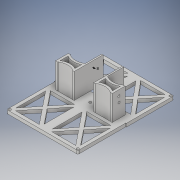
# Autodesk Inventor part: 4 Tape Measure Holder 2 Lid
Saved by Autodesk Inventor 2019 (Build 230136000, 136)
## iProperties
Created: 2019-01-05
Part Number: 4 Tape Measure Holder 2 Lid
Material: Generic
Document SubType Name: Modeling
Designer: ashle
Density: 1 g/cm^3
Appearance: Default
sut: 4.300 mm
TMROL: 45.000 mm
AW: 4.000 mm
WD: 50.000 mm
WW: 20.000 mm
sh: 4.000 mm
BSHH: 10.000 mm
Author: ashle
Autodesk Inventor part; units mm, degrees
ref_plane "YZ Plane" through (0, 0, 0) normal (1, 0, 0) x (0, 1, 0)
ref_plane "XZ Plane" through (0, 0, 0) normal (0, 1, 0) x (-1, 0, 0)
ref_plane "XY Plane" through (0, 0, 0) normal (0, 0, 1) x (1, 0, 0)
sketch "Main Body Sketch" plane through (0, 0, 0) normal (0, 1, 0) x (-1, 0, 0)
  line L0 (162.9728, 0) -> (-170.7717, 0) construction
  line L1 (0, -112.4599) -> (0, 110.3364) construction
  line L2 (65, -85.25) -> (-65, -85.25)
  line L3 (-65, -85.25) -> (-65, 0)
  line L4 (-65, 0) -> (65, 0)
  line L5 (65, 0) -> (65, -85.25)
  line L6 (64, 0) -> (-64, 0)
  line L7 (-64, 0) -> (-64, 86.25)
  line L8 (-64, 86.25) -> (64, 86.25)
  line L9 (64, 86.25) -> (64, 0)
  line L10 (7.5, -85.25) -> (-7.5, -85.25)
  line L11 (-7.5, -85.25) -> (-7.5, 86.25) construction
  line L12 (-7.5, 86.25) -> (7.5, 86.25)
  line L13 (7.5, 86.25) -> (7.5, -85.25) construction
  line L14 (65, -11.5) -> (-65, -11.5) construction
  line L15 (-65, -11.5) -> (-65, 0) construction
  line L16 (-65, 0) -> (65, 0) construction
  line L17 (65, 0) -> (65, -11.5) construction
  line L18 (64, 0) -> (-64, 0)
  line L19 (-64, 0) -> (-64, 11.5) construction
  line L20 (-64, 11.5) -> (64, 11.5) construction
  line L21 (64, 11.5) -> (64, 0) construction
  line L22 (59, -79.25) -> (7.5, -79.25) construction
  line L23 (7.5, -79.25) -> (7.5, -17.5) construction
  line L24 (7.5, -17.5) -> (59, -17.5) construction
  line L25 (59, -17.5) -> (59, -79.25) construction
  line L26 (-7.5, -79.25) -> (-59, -79.25) construction
  line L27 (-59, -79.25) -> (-59, -17.5) construction
  line L28 (-59, -17.5) -> (-7.5, -17.5) construction
  line L29 (-7.5, -17.5) -> (-7.5, -79.25) construction
  line L30 (58, 17.5) -> (7.5, 17.5) construction
  line L31 (7.5, 17.5) -> (7.5, 80.25) construction
  line L32 (7.5, 80.25) -> (58, 80.25) construction
  line L33 (58, 80.25) -> (58, 17.5) construction
  line L34 (-7.5, 17.5) -> (-58, 17.5) construction
  line L35 (-58, 17.5) -> (-58, 80.25) construction
  line L36 (-58, 80.25) -> (-7.5, 80.25) construction
  line L37 (-7.5, 80.25) -> (-7.5, 17.5) construction
  line L38 (59, -79.25) -> (7.5, -17.5) construction
  line L39 (7.5, -79.25) -> (59, -17.5) construction
  line L40 (58, 17.5) -> (7.5, 80.25) construction
  line L41 (7.5, 17.5) -> (58, 80.25) construction
  line L42 (55.6629, 15.6191) -> (60.3371, 19.3809) construction
  line L43 (60.3371, 19.3809) -> (9.8371, 82.1309) construction
  line L44 (9.8371, 82.1309) -> (5.1629, 78.3691) construction
  line L45 (5.1629, 78.3691) -> (55.6629, 15.6191) construction
  line L46 (61.3039, -77.3285) -> (56.6961, -81.1715) construction
  line L47 (56.6961, -81.1715) -> (5.1961, -19.4215) construction
  line L48 (5.1961, -19.4215) -> (9.8039, -15.5785) construction
  line L49 (9.8039, -15.5785) -> (61.3039, -77.3285) construction
  line L50 (9.8039, -81.1715) -> (5.1961, -77.3285) construction
  line L51 (5.1961, -77.3285) -> (56.6961, -15.5785) construction
  line L52 (56.6961, -15.5785) -> (61.3039, -19.4215) construction
  line L53 (61.3039, -19.4215) -> (9.8039, -81.1715) construction
  line L54 (9.8371, 15.6191) -> (5.1629, 19.3809) construction
  line L55 (5.1629, 19.3809) -> (55.6629, 82.1309) construction
  line L56 (55.6629, 82.1309) -> (60.3371, 78.3691) construction
  line L57 (60.3371, 78.3691) -> (9.8371, 15.6191) construction
  line L58 (33.25, -43.6911) -> (55.0936, -17.5)
  line L59 (55.0936, -17.5) -> (11.4064, -17.5)
  line L60 (11.4064, -17.5) -> (33.25, -43.6911)
  line L61 (54.1491, 17.5) -> (32.75, 44.09)
  line L62 (32.75, 44.09) -> (11.3509, 17.5)
  line L63 (11.3509, 17.5) -> (54.1491, 17.5)
  line L64 (58, 22.285) -> (58, 75.465)
  line L65 (58, 75.465) -> (36.6009, 48.875)
  line L66 (36.6009, 48.875) -> (58, 22.285)
  line L67 (32.75, 53.66) -> (54.1491, 80.25)
  line L68 (54.1491, 80.25) -> (11.3509, 80.25)
  line L69 (11.3509, 80.25) -> (32.75, 53.66)
  line L70 (7.5, 22.285) -> (28.8991, 48.875)
  line L71 (28.8991, 48.875) -> (7.5, 75.465)
  line L72 (7.5, 75.465) -> (7.5, 22.285)
  line L73 (59, -74.5661) -> (59, -22.1839)
  line L74 (59, -22.1839) -> (37.1564, -48.375)
  line L75 (37.1564, -48.375) -> (59, -74.5661)
  line L76 (55.0936, -79.25) -> (33.25, -53.0589)
  line L77 (33.25, -53.0589) -> (11.4064, -79.25)
  line L78 (11.4064, -79.25) -> (55.0936, -79.25)
  line L79 (7.5, -74.5661) -> (29.3436, -48.375)
  line L80 (29.3436, -48.375) -> (7.5, -22.1839)
  line L81 (7.5, -22.1839) -> (7.5, -74.5661)
  line L82 (-59, -79.25) -> (-7.5, -79.25) construction
  line L83 (-7.5, -79.25) -> (-7.5, -17.5) construction
  line L84 (-7.5, -17.5) -> (-59, -17.5) construction
  line L85 (-59, -17.5) -> (-59, -79.25) construction
  line L86 (-59, -79.25) -> (-7.5, -17.5) construction
  line L87 (-7.5, -79.25) -> (-59, -17.5) construction
  line L88 (-61.3039, -77.3285) -> (-56.6961, -81.1715) construction
  line L89 (-56.6961, -81.1715) -> (-5.1961, -19.4215) construction
  line L90 (-5.1961, -19.4215) -> (-9.8039, -15.5785) construction
  line L91 (-9.8039, -15.5785) -> (-61.3039, -77.3285) construction
  line L92 (-9.8039, -81.1715) -> (-5.1961, -77.3285) construction
  line L93 (-5.1961, -77.3285) -> (-56.6961, -15.5785) construction
  line L94 (-56.6961, -15.5785) -> (-61.3039, -19.4215) construction
  line L95 (-61.3039, -19.4215) -> (-9.8039, -81.1715) construction
  line L96 (-33.25, -43.6911) -> (-55.0936, -17.5)
  line L97 (-55.0936, -17.5) -> (-11.4064, -17.5)
  line L98 (-11.4064, -17.5) -> (-33.25, -43.6911)
  line L99 (-59, -74.5661) -> (-59, -22.1839)
  line L100 (-59, -22.1839) -> (-37.1564, -48.375)
  line L101 (-37.1564, -48.375) -> (-59, -74.5661)
  line L102 (-55.0936, -79.25) -> (-33.25, -53.0589)
  line L103 (-33.25, -53.0589) -> (-11.4064, -79.25)
  line L104 (-11.4064, -79.25) -> (-55.0936, -79.25)
  line L105 (-7.5, -74.5661) -> (-29.3436, -48.375)
  line L106 (-29.3436, -48.375) -> (-7.5, -22.1839)
  line L107 (-7.5, -22.1839) -> (-7.5, -74.5661)
  line L108 (-58, 17.5) -> (-7.5, 17.5) construction
  line L109 (-7.5, 17.5) -> (-7.5, 80.25) construction
  line L110 (-7.5, 80.25) -> (-58, 80.25) construction
  line L111 (-58, 80.25) -> (-58, 17.5) construction
  line L112 (-58, 17.5) -> (-7.5, 80.25) construction
  line L113 (-7.5, 17.5) -> (-58, 80.25) construction
  line L114 (-55.6629, 15.6191) -> (-60.3371, 19.3809) construction
  line L115 (-60.3371, 19.3809) -> (-9.8371, 82.1309) construction
  line L116 (-9.8371, 82.1309) -> (-5.1629, 78.3691) construction
  line L117 (-5.1629, 78.3691) -> (-55.6629, 15.6191) construction
  line L118 (-9.8371, 15.6191) -> (-5.1629, 19.3809) construction
  line L119 (-5.1629, 19.3809) -> (-55.6629, 82.1309) construction
  line L120 (-55.6629, 82.1309) -> (-60.3371, 78.3691) construction
  line L121 (-60.3371, 78.3691) -> (-9.8371, 15.6191) construction
  line L122 (-54.1491, 17.5) -> (-32.75, 44.09)
  line L123 (-32.75, 44.09) -> (-11.3509, 17.5)
  line L124 (-11.3509, 17.5) -> (-54.1491, 17.5)
  line L125 (-58, 22.285) -> (-58, 75.465)
  line L126 (-58, 75.465) -> (-36.6009, 48.875)
  line L127 (-36.6009, 48.875) -> (-58, 22.285)
  line L128 (-32.75, 53.66) -> (-54.1491, 80.25)
  line L129 (-54.1491, 80.25) -> (-11.3509, 80.25)
  line L130 (-11.3509, 80.25) -> (-32.75, 53.66)
  line L131 (-7.5, 22.285) -> (-28.8991, 48.875)
  line L132 (-28.8991, 48.875) -> (-7.5, 75.465)
  line L133 (-7.5, 75.465) -> (-7.5, 22.285)
  line L134 (71.3038, -11) -> (3.6263, -11) construction
  line L135 (71.3038, -7) -> (3.6263, -7) construction
  line L136 (47, -13.6904) -> (47, -1.8887) construction
  line L137 (20, -13.6904) -> (20, -1.8887) construction
  line L138 (47, -11.5) -> (20, -11.5)
  line L139 (20, -11.5) -> (20, -11)
  line L140 (47, -11.5) -> (47, -11)
  line L141 (33.5, -14.616) -> (33.5, -1.8887) construction
  arc A0 (47, -11) -> (20, -11) centre (33.5, -31.7812) ccw
  line L142 (-47, -13.6904) -> (-47, -1.8887) construction
  line L143 (-20, -13.6904) -> (-20, -1.8887) construction
  line L144 (-47, -11.5) -> (-20, -11.5)
  line L145 (-20, -11.5) -> (-20, -11)
  line L146 (-47, -11.5) -> (-47, -11)
  arc A1 (-20, -11) -> (-47, -11) centre (-33.5, -31.7812) ccw
  line L147 (47, 13.6904) -> (47, 1.8887) construction
  line L148 (20, 13.6904) -> (20, 1.8887) construction
  line L149 (47, 11.5) -> (20, 11.5)
  line L150 (20, 11.5) -> (20, 11)
  line L151 (47, 11.5) -> (47, 11)
  line L152 (33.5, 14.616) -> (33.5, 1.8887) construction
  arc A2 (20, 11) -> (47, 11) centre (33.5, 31.7812) ccw
  line L153 (-47, 11.5) -> (-20, 11.5)
  line L154 (-47, 11.5) -> (-47, 11)
  line L155 (-20, 11.5) -> (-20, 11)
  arc A3 (-47, 11) -> (-20, 11) centre (-33.5, 31.7812) ccw
  line L156 (-47, 13.6904) -> (-47, 1.8887) construction
  line L157 (-20, 13.6904) -> (-20, 1.8887) construction
  point P0 (-33.5, -1.8887)
  point P1 (3.6263, 11)
  point P2 (3.6263, 7)
  point P3 (-33.5, 1.8887)
  dimension "d19" = 130
  dimension "d20" = 128
  dimension "d21" = 86.25
  dimension "d22" = 85.25
  dimension "d23" = 65
  dimension "d24" = 64
  dimension "d25" = 15
  dimension "d26" = 7.5
  dimension "d27" = 11.5
  dimension "d28" = 11.5
  dimension "d29" = 6
  dimension "d30" = 6
  dimension "d31" = 6
  dimension "d32" = 6
  dimension "d33" = 6
  dimension "d34" = 6
  dimension "d35" = 6
  dimension "d36" = 6
  dimension "d37" = 6
  dimension "d38" = 6
  dimension "d39" = 6
  dimension "d40" = 6
  dimension "d41" = 6
  dimension "d42" = 6
  dimension "d43" = 6
  dimension "d44" = 6
  dimension "d45" = 0.5
  dimension "d46" = 4
  dimension "d47" = 27
  dimension "d48" = 20
  dimension "d49" = 27
  dimension "d50" = 40
  constraints: 318 end point, 75 symmetric about line, 38 collinear, 30 parallel, 25 point on line, 14 horizontal, 14 perpendicular, 8 midpoint, 8 point on circle, 6 vertical, 4 centre point, 1 tangent, 3 other
  measures "d19" distance of L2.start L2.end
  measures "d20" distance of L7.end L8.end
  measures "d21" distance of L8.end L6.start
  measures "d22" distance of L4.end L2.start
  measures "d23" distance between parallel lines of L1 L5
  measures "d24" distance between parallel lines of L9 L1
  measures "d25" distance between parallel lines of L11 L13
  measures "d26" distance between parallel lines of L1 L11
  measures "d27" distance between parallel lines of L0 L20
  measures "d28" distance between parallel lines of L14 L0
  measures "d29" distance between parallel lines of L2 L22
  measures "d30" distance between parallel lines of L2 L26
  measures "d31" distance between parallel lines of L14 L28
  measures "d32" distance between parallel lines of L3 L27
  measures "d33" distance between parallel lines of L5 L25
  measures "d34" distance between parallel lines of L14 L24
  measures "d35" distance between parallel lines of L20 L30
  measures "d36" distance between parallel lines of L9 L33
  measures "d37" distance between parallel lines of L8 L32
  measures "d38" distance between parallel lines of L7 L35
  measures "d39" distance between parallel lines of L20 L34
  measures "d40" distance between parallel lines of L8 L36
  measures "d41" distance between parallel lines of L45 L43
  measures "d42" distance between parallel lines of L55 L57
  measures "d43" distance between parallel lines of L47 L49
  measures "d44" distance between parallel lines of L51 L53
  measures "d45" distance between parallel lines of L14 L134
  measures "d46" distance between parallel lines of L134 L135
  measures "d47" distance between parallel lines of L137 L136
  measures "d48" distance between parallel lines of L1 L137
  measures "d49" diameter of L137 L141
  measures "d50" distance between parallel lines of L143 L137
extrude "Main Body Extrusion" add sketch "Main Body Sketch" along normal blind 6
sketch "TMS ROLL OUT" plane through (0, 6, 0) normal (0, 1, 0) x (1, 0, 0)
  line L0 (-47, 11) -> (-47, 11.5)
  line L1 (-20, 11.5) -> (-20, 11) projected
  line L2 (-20, 11.5) -> (-20, 11)
  arc A0 (-47, 11) -> (-20, 11) centre (-33.5, 31.7812) ccw
  line L3 (20, 11.5) -> (20, 11) projected
  line L4 (20, 11) -> (20, 11.5)
  line L5 (47, 11.5) -> (47, 11) projected
  line L6 (47, 11.5) -> (47, 11)
  arc A1 (20, 11) -> (47, 11) centre (33.5, 31.7812) ccw
  arc A2 (47, -11) -> (20, -11) centre (33.5, -31.7812) ccw projected
  line L7 (20, -11) -> (20, -11.5)
  line L8 (47, -11.5) -> (47, -11) projected
  line L9 (47, -11.5) -> (47, -11)
  arc A3 (47, -11) -> (20, -11) centre (33.5, -31.7812) ccw
  line L10 (-47, -11.5) -> (-47, -11) projected
  line L11 (-47, -11) -> (-47, -11.5)
  line L12 (-20, -11) -> (-20, -11.5) projected
  line L13 (-20, -11.5) -> (-20, -11)
  arc A4 (-20, -11) -> (-47, -11) centre (-33.5, -31.7812) ccw
  line L14 (-47, 11.5) -> (-51, 11.5)
  line L15 (-51, 11.5) -> (-51, -11.5)
  line L16 (-51, -11.5) -> (-47, -11.5)
  line L17 (-47, 11.5) -> (-20, 11.5) construction
  line L18 (-20, -11.5) -> (-47, -11.5) construction
  line L19 (-17.5, 11.5) -> (-20, 11.5)
  line L20 (-20, -11.5) -> (-17.5, -11.5)
  line L21 (-17.5, -11.5) -> (-17.5, 11.5)
  line L22 (20, 11.5) -> (17.5, 11.5)
  line L23 (17.5, 11.5) -> (17.5, -11.5)
  line L24 (17.5, -11.5) -> (20, -11.5)
  line L25 (47, 11.5) -> (51, 11.5)
  line L26 (51, 11.5) -> (51, -11.5)
  line L27 (51, -11.5) -> (47, -11.5)
  line L28 (20, 11.5) -> (47, 11.5) construction
  line L29 (47, -11.5) -> (20, -11.5) construction
  point P0 (0, 0)
  dimension "d53" = 24.7812
  dimension "d54" = 24.7812
  dimension "d55" = 24.7812
  dimension "d56" = 24.7812
  dimension "d57" = 4
  dimension "d60" = 4
  dimension "d90" = 35
  constraints: 40 end point, 9 collinear, 8 point on circle, 7 equal length, 4 centre point, 4 horizontal, 3 perpendicular, 3 vertical
  measures "d53" radius of A0
  measures "d54" radius of A1
  measures "d55" radius of A3
  measures "d56" radius of A4
  measures "d57" distance between parallel lines of L15 L0
  measures "d60" distance between parallel lines of L5 L26
  measures "d90" distance between parallel lines of L21 L23
extrude "TM Roll Out" add sketch "TMS ROLL OUT" along normal blind 45
sketch "Sketch3" plane through (0, 51, 0) normal (0, 1, 0) x (1, 0, 0)
  line L0 (47, -15.7755) -> (47, 16.2908) construction
  line L1 (47, -11) -> (47, -11.5) projected
  line L2 (20, -14.3518) -> (20, 15.2061) construction
  line L3 (20, -11.5) -> (20, -11) projected
  line L4 (47, 11.5) -> (47, 11) construction
  line L5 (20, 11) -> (20, 11.5) construction
  arc A0 (47, -7.1416) -> (21.5, -5.9813) centre (33.2845, -27.7812) ccw
  arc A1 (47, -11) -> (20, -11) centre (33.5, -31.7812) ccw projected
  line L6 (67.0772, 0) -> (9.1406, 0) construction
  arc A2 (21.5, 5.9813) -> (47, 7.1416) centre (33.2845, 27.7812) ccw
  line L7 (47, -7.1416) -> (47, 7.1416)
  line L8 (21.5, -5.9813) -> (21.5, 5.9813)
  line L9 (51, -11.5) -> (51, 11.5) projected
  line L10 (17.5, 11.5) -> (17.5, -11.5) projected
  line L11 (0, -27.7812) -> (0, 31.8855) construction
  line L12 (-47, -11) -> (-47, -11.5)
  line L13 (-20, -11.5) -> (-20, -11)
  line L14 (-47, 11.5) -> (-47, 11) construction
  line L15 (-20, 11) -> (-20, 11.5) construction
  arc A3 (-21.5, -5.9813) -> (-47, -7.1416) centre (-33.2845, -27.7812) ccw
  arc A4 (-20, -11) -> (-47, -11) centre (-33.5, -31.7812) ccw
  arc A5 (-47, 7.1416) -> (-21.5, 5.9813) centre (-33.2845, 27.7812) ccw
  line L16 (-47, -7.1416) -> (-47, 7.1416)
  line L17 (-21.5, -5.9813) -> (-21.5, 5.9813)
  line L18 (-51, -11.5) -> (-51, 11.5)
  line L19 (-17.5, 11.5) -> (-17.5, -11.5)
  point P0 (0, 0)
  point P1 (-47, -15.7755)
  point P2 (-20, -14.3518)
  dimension "d65" = 24.7812
  dimension "d66" = 4
  dimension "d67" = 4
  dimension "d68" = 4
  constraints: 28 end point, 24 symmetric about line, 10 point on circle, 5 centre point, 4 collinear, 4 vertical, 1 horizontal, 1 parallel, 4 other
  measures "d65" radius of A0
  measures "d66" vertical distance of A0.centre A1.centre
  measures "d67" distance between parallel lines of L9 L7
  measures "d68" distance between parallel lines of L10 L8
extrude "Center Swissing" cut sketch "Sketch3" against normal up to surface (51 mm away)
sketch "Sketch4" plane through (0, 6, 0) normal (0, 1, 0) x (1, 0, 0)
  line L0 (-65, 85.25) -> (-59, 85.25) construction
  line L1 (-59, 85.25) -> (-59, 79.25) construction
  line L2 (-59, 79.25) -> (-65, 79.25) construction
  line L3 (-65, 79.25) -> (-65, 85.25) construction
  line L4 (65, 85.25) -> (-65, 85.25) construction
  line L5 (-65, 85.25) -> (-65, 0) construction
  line L6 (-59, 22.1839) -> (-59, 74.5661) construction
  line L7 (-55.0936, 79.25) -> (-11.4064, 79.25) construction
  circle A0 centre (-62, 82.25) radius 2.15
  line L8 (-62, 82.25) -> (-62, 85.25) construction
  line L9 (-65, 85.25) -> (65, 85.25) construction
  line L10 (-62, 82.25) -> (-62, 79.25) construction
  line L11 (-62, 82.25) -> (-59, 82.25) construction
  line L12 (-62, 82.25) -> (-65, 82.25) construction
  line L13 (-65, 0) -> (-65, 85.25) construction
  line L14 (0, 94.5272) -> (0, -100.1402) construction
  line L15 (65, 85.25) -> (59, 85.25) construction
  line L16 (59, 85.25) -> (59, 79.25) construction
  line L17 (59, 79.25) -> (65, 79.25) construction
  line L18 (65, 79.25) -> (65, 85.25) construction
  circle A1 centre (62, 82.25) radius 2.15
  line L19 (62, 82.25) -> (62, 85.25) construction
  line L20 (62, 82.25) -> (62, 79.25) construction
  line L21 (62, 82.25) -> (59, 82.25) construction
  line L22 (62, 82.25) -> (65, 82.25) construction
  line L23 (-64, -86.25) -> (-58, -86.25) construction
  line L24 (-58, -86.25) -> (-58, -80.25) construction
  line L25 (-58, -80.25) -> (-64, -80.25) construction
  line L26 (-64, -80.25) -> (-64, -86.25) construction
  line L27 (-11.3509, -80.25) -> (-54.1491, -80.25) construction
  line L28 (-58, -75.465) -> (-58, -22.285) construction
  line L29 (-64, -86.25) -> (64, -86.25) construction
  line L30 (-64, 0) -> (-64, -86.25) construction
  circle A2 centre (-61, -83.25) radius 2.15
  line L31 (-61, -83.25) -> (-61, -80.25) construction
  line L32 (-61, -83.25) -> (-61, -86.25) construction
  line L33 (64, -86.25) -> (-64, -86.25) construction
  line L34 (-61, -83.25) -> (-64, -83.25) construction
  line L35 (-61, -83.25) -> (-58, -83.25) construction
  line L36 (64, -86.25) -> (58, -86.25) construction
  line L37 (58, -86.25) -> (58, -80.25) construction
  line L38 (58, -80.25) -> (64, -80.25) construction
  line L39 (64, -80.25) -> (64, -86.25) construction
  circle A3 centre (61, -83.25) radius 2.15
  line L40 (61, -83.25) -> (61, -80.25) construction
  line L41 (61, -83.25) -> (61, -86.25) construction
  line L42 (61, -83.25) -> (64, -83.25) construction
  line L43 (61, -83.25) -> (58, -83.25) construction
  circle A4 centre (0, 0) radius 2.15
  dimension "d71" = 4.3
  dimension "d72" = 4.3
  dimension "d73" = 4.3
  constraints: 66 end point, 20 symmetric about line, 12 collinear, 9 point on line, 5 centre point, 5 midpoint, 5 perpendicular, 4 parallel, 2 horizontal, 2 vertical, 1 coincident, 2 other
  measures "d71" diameter of A0
  measures "d72" diameter of A2
  measures "d73" diameter of A4
extrude "Screw Holes Cut" cut sketch "Sketch4" against normal up to surface (6 mm away)
fillet "Fillet2" radius 2 4 edges at (-64, 3, 86.25) (-65, 3, -85.25) (65, 3, -85.25) (64, 3, 86.25)
ref_plane "Work Plane1" through (51, 6, 9.5) normal (1, 0, 0) x (0, 0, -1)
sketch "Sketch5" plane through (51, 6, 9.5) normal (1, 0, 0) x (0, 0, -1)
  circle A0 centre (9.8855, 35) radius 2
  circle A1 centre (10.1251, 25.0029) radius 2
  line L0 (-2, 45) -> (21, 45) projected
  line L1 (10.1251, 25.0029) -> (-0.2499, 25.0029) construction
  line L2 (9.8855, 35) -> (-0.7289, 35) construction
  line L3 (9.8855, 35) -> (20.5, 35) construction
  line L4 (20.5, -6) -> (20.5, 45) construction
  line L5 (10.1251, 25.0029) -> (20.5, 25.0029) construction
  dimension "d78" = 4
  dimension "d79" = 4
  dimension "d88" = 10
  dimension "d91" = 10
  constraints: 8 end point, 3 horizontal, 2 centre point, 2 collinear, 2 point on line, 1 perpendicular
  measures "d78" diameter of A0
  measures "d79" diameter of A1
  measures "d88" distance of L2.start L1.start
  measures "d91" distance from line of L0 L2.start
extrude "Side Screw holes" cut sketch "Sketch5" against normal up to surface (4 mm away)
ref_plane "Work Plane3" through (0, 6, -11.5) normal (-1, 0, 0) x (0, 0, 1)
mirror "Mirror1" about plane through (0, 6, -11.5) normal (-1, 0, 0) of "Side Screw holes"
sketch "Sketch7" plane through (-17.5, 6, -11.5) normal (0, 0, -1) x (-1, 0, 0)
  line L0 (2.5, 0) -> (0, 0)
  line L1 (0, 0) -> (0, 45)
  line L2 (0, 45) -> (2.5, 45)
  line L3 (2.5, 45) -> (2.5, 0)
  line L4 (-35, 0) -> (-37.5, 0)
  line L5 (-37.5, 0) -> (-37.5, 45)
  line L6 (-37.5, 45) -> (-35, 45)
  line L7 (-35, 45) -> (-35, 0)
  line L8 (0, 0) -> (0, 45) projected
  line L9 (2.5, 0) -> (2.5, 45) projected
  line L10 (2.5, 0) -> (0, 0) projected
  line L11 (-35, 0) -> (-37.5, 0) projected
  line L12 (-35, 0) -> (-35, 45) projected
  line L13 (-37.5, 0) -> (-37.5, 45) projected
  line L14 (-37.5, 45) -> (-35, 45) projected
  line L15 (0, 45) -> (2.5, 45) projected
  point P0 (-17.5, -6)
  constraints: 16 end point, 8 collinear, 4 parallel, 2 horizontal, 2 perpendicular
extrude "Extrusion7" add sketch "Sketch7" along normal blind 29
sketch "Sketch8" plane through (-20, 0, -11.5) normal (-1, 0, 0) x (0, 0, 1)
  circle A0 centre (-14.9868, 36.4736) radius 4
  point P0 (11.5, 0)
  dimension "d96" = 8
  constraints: 1 centre point
  measures "d96" diameter of A0
equation "\"d19\" = TM1THL"
equation "\"d20\" = TM2THL"
equation "\"d21\" = TM2TVL"
equation "\"d22\" = TM1TVL"
equation "\"d23\" = 0.5 * TM1THL"
equation "\"d24\" = 0.5 * TM2THL"
equation "\"d25\" = HS"
equation "\"d26\" = 0.5 * HS"
equation "\"d27\" = 0.5 * ArcBH"
equation "\"d28\" = 0.5 * ArcBH"
equation "\"d29\" = uw"
equation "\"d30\" = uw"
equation "\"d31\" = uw"
equation "\"d32\" = uw"
equation "\"d33\" = uw"
equation "\"d34\" = uw"
equation "\"d35\" = uw"
equation "\"d36\" = uw"
equation "\"d37\" = uw"
equation "\"d38\" = uw"
equation "\"d39\" = uw"
equation "\"d40\" = uw"
equation "\"d41\" = uw"
equation "\"d42\" = uw"
equation "\"d43\" = uw"
equation "\"d44\" = uw"
equation "\"d45\" = ArcEH"
equation "\"d46\" = ArcH"
equation "\"d47\" = ArcW"
equation "\"d48\" = 0.5 * ArcDB"
equation "\"d49\" = ArcW"
equation "\"d51\" = uw"
equation "\"d53\" = ArcR"
equation "\"d54\" = ArcR"
equation "\"d55\" = ArcR"
equation "\"d56\" = ArcR"
equation "\"d57\" = AW"
equation "\"d60\" = AW"
equation "\"d63\" = TMROL"
equation "\"d65\" = ArcR"
equation "\"d71\" = sut"
equation "\"d72\" = sut"
equation "\"d73\" = sut"
equation "\"d78\" = sh"
equation "\"d79\" = sh"
equation "\"d88\" = BSHH"
equation "\"AW\" = 4"
equation "\"WD\" = 50"
equation "\"WW\" = 20"
equation "\"sut\" = 4.3"
equation "\"sh\" = 4"
equation "\"BSHH\" = 10"
equation "\"CHexW\" = 34.5"
equation "\"TM1THL\" = 130"
equation "\"TM2THL\" = 128"
equation "\"TM2TVL\" = 86.25"
equation "\"TM1TVL\" = 85.25"
equation "\"HS\" = 15"
equation "\"ArcBH\" = 23"
equation "\"uw\" = 6"
equation "\"ArcEH\" = 0.5"
equation "\"ArcH\" = 4"
equation "\"ArcW\" = 27"
equation "\"ArcDB\" = 40"
equation "\"ArcR\" = 24.78125"
equation "\"TMROL\" = 45"
body "Solid1"
